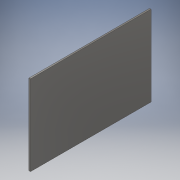
# Autodesk Inventor part: LongTLeftRightOutRev3
Saved by Autodesk Inventor 2017 (Build 210142000, 142)
## iProperties
Created: 2016-12-13
Part Number: LongTLeftRightOutRev3
Material: Steel, Mild
Document SubType Name: Sheet Metal
Designer: Robert.Chapman
Density: 7.85 g/cm^3
Sheet Metal Rule: Default
Appearance: Semi-Polished
Author: Robert.Chapman
Autodesk Inventor part; units mm, degrees
ref_plane "YZ Plane" through (0, 0, 0) normal (1, 0, 0) x (0, 1, 0)
ref_plane "XZ Plane" through (0, 0, 0) normal (0, 1, 0) x (-1, 0, 0)
ref_plane "XY Plane" through (0, 0, 0) normal (0, 0, 1) x (1, 0, 0)
sketch "Sketch1" plane through (0, 0, 0) normal (1, 0, 0) x (0, 1, 0)
  line L0 (-127, 190.5) -> (127, 190.5)
  line L1 (127, 190.5) -> (127, -190.5)
  line L2 (127, -190.5) -> (-127, -190.5)
  line L3 (-127, -190.5) -> (-127, 190.5)
  line L4 (-127, 190.5) -> (127, -190.5) construction
  line L5 (127, 190.5) -> (-127, -190.5) construction
  point P0 (0, 0)
  dimension "d0" = 381
  dimension "d1" = 254
  measures "d0" distance of L0.end L1.end
  measures "d1" distance of L0.start L0.end
extrude "Plate1" add sketch "Sketch1" along normal blind 4.7625
equation "\"BendRadius\" = Thickness"
equation "\"BendReliefWidth\" = Thickness"
equation "\"BendReliefDepth\" = 0.5 * Thickness"
equation "\"CornerReliefSize\" = 4 * Thickness"
equation "\"MinimumRemnant\" = 2 * Thickness"
equation "\"TransitionRadius\" = BendRadius"
equation "\"JacobiRadiusSize\" = BendRadius"
equation "\"GapSize\" = Thickness"
equation "\"d2\" = BendRadius"
equation "\"Thickness\" = 4.7625"
body "Solid1"
